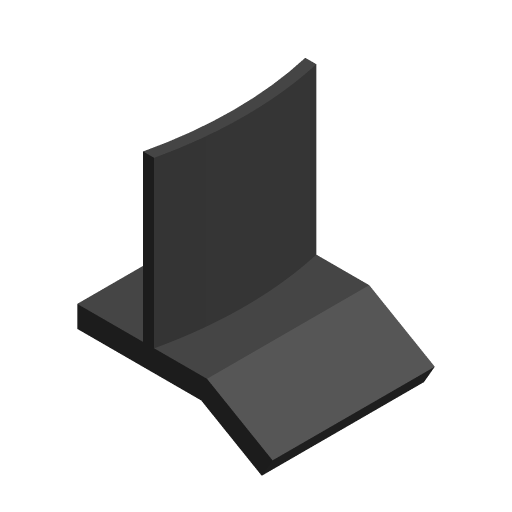
# Autodesk Inventor part: Camera retention
Saved by Autodesk Inventor 2024 (Build 280153000, 153)
## iProperties
Part Number: Camera retention
Material: Generic
Document SubType Name: Modeling
Designer: Jamie
Appearance: Default
Author: Jamie
Autodesk Inventor part; units mm, degrees
ref_plane "YZ Plane" through (0, 0, 0) normal (1, 0, 0) x (0, 1, 0)
ref_plane "XZ Plane" through (0, 0, 0) normal (0, 1, 0) x (-1, 0, 0)
ref_plane "XY Plane" through (0, 0, 0) normal (0, 0, 1) x (1, 0, 0)
sketch "Sketch3" plane through (0, 0, 0) normal (0, 1, 0) x (-1, 0, 0)
  circle A0 centre (0, 0) radius 33
  circle A1 centre (0, 0) radius 34
  line L0 (-30.4296, 7.5) -> (-38.9548, 7.5)
  line L1 (-38.9548, 7.5) -> (-38.9548, -7.5)
  line L2 (-38.9548, -7.5) -> (-30.4296, -7.5)
  line L3 (-30.4296, -7.5) -> (-30.4296, 7.5)
  point P0 (-33.1625, -7.5)
  point P1 (-32.1364, -7.5)
  point P2 (-32.1364, 7.5)
  point P3 (-33.1625, 7.5)
  dimension "d9" = 66
  dimension "d10" = 68
  dimension "d11" = 7.5
  dimension "d12" = 7.5
  constraints: 8 end point, 2 centre point, 2 coincident, 2 parallel, 1 horizontal, 1 perpendicular
  measures "d9" diameter of A0
  measures "d10" diameter of A1
  measures "d11" distance from line of point (0, 0) L0
  measures "d12" distance from line of point (0, 0) L2
extrude "Extrusion2" add sketch "Sketch3" along normal blind 15.25 contours A0 L2 A1 L0 picked at (-32.7342, -5.8399)
sketch "Sketch4" plane through (0, 0, 0) normal (0, -1, 0) x (1, 0, 0)
  line L0 (26.0495, 7.5) -> (38.0495, 7.5)
  line L1 (38.0495, 7.5) -> (38.0495, -7.5)
  line L2 (38.0495, -7.5) -> (26.0495, -7.5)
  line L3 (26.0495, -7.5) -> (26.0495, 7.5)
  line L4 (33.1625, -7.5) -> (32.1364, -7.5) projected
  line L5 (32.1364, 7.5) -> (33.1625, 7.5) projected
  point P0 (0, 0)
  point P1 (32.6495, -7.5)
  point P2 (32.6495, -7.5)
  dimension "d15" = 6.6
  dimension "d16" = 5.4
  dimension "d17" = 0
  dimension "d18" = 0
  constraints: 8 end point, 2 midpoint, 2 parallel, 1 horizontal, 1 perpendicular
  measures "d15" distance from line of L3 point (32.649, -7.5)
  measures "d16" distance from line of point (32.649, -7.5) L1
  measures "d17" distance between parallel lines of L4 L2
  measures "d18" distance between parallel lines of L5 L0
extrude "Extrusion3" add sketch "Sketch4" along normal blind 2
sketch "Sketch5" plane through (0, -2, 0) normal (0, -1, 0) x (1, 0, 0)
  circle A0 centre (29.0005, 0) radius 2
  line L0 (38.0495, 7.5) -> (26.0495, 7.5) projected
  line L1 (32.1364, 7.5) -> (33.1625, 7.5) projected
  point P0 (0, 0)
  point P1 (32.6495, 7.5)
  dimension "d21" = 4
  dimension "d22" = 7.5
  dimension "d23" = 3.649
  constraints: 1 centre point, 1 midpoint
  measures "d21" diameter of A0
  measures "d22" distance from line of L0 A0.centre
  measures "d23" horizontal distance of point (32.649, 7.5) A0.centre
extrude "Extrusion4" cut sketch "Sketch5" against normal blind 2
ref_plane "Work Plane1" through (38.0495, 0, -7.5) normal (0.5, 0.8660254, 0) x (0, 0, 1)
sketch "Sketch6" plane through (38.0495, 0, -7.5) normal (0.5, 0.8660254, 0) x (0, 0, 1)
  line L0 (15, 0) -> (0, 0)
  line L1 (0, 0) -> (0, 7)
  line L2 (0, 7) -> (15, 7)
  line L3 (15, 7) -> (15, 0)
  line L4 (0, 0) -> (15, 0) projected
  line L5 (15, 0) -> (15, -4.2322) projected
  line L6 (0, -4.2322) -> (0, 0) projected
  point P0 (7.5, -32.9518)
  point P1 (15, 3.5)
  dimension "d27" = 0
  dimension "d28" = 0
  dimension "d29" = 0
  dimension "d30" = 7
  constraints: 8 end point, 2 parallel, 1 horizontal, 1 midpoint, 1 perpendicular
  measures "d27" distance between parallel lines of L4 L0
  measures "d28" distance from line of L5 point (15, 3.5)
  measures "d29" distance between parallel lines of L6 L1
  measures "d30" distance of L0.end L1.end
extrude "Extrusion5" add sketch "Sketch6" against normal blind 2
sketch "Sketch7" plane through (37.0495, -1.7321, -7.5) normal (-0.5, -0.8660254, 0) x (0.8660254, -0.5, 0)
  circle A0 centre (5.0359, 4.5) radius 1
  circle A1 centre (5.0359, 10.5) radius 1
  ellipse E0 centre (-7.8367, 7.5) end of major axis (-7.8367, 9.5) minor radius 1.7321 projected
  line L0 (0.5359, 0) -> (0.5359, 15) projected
  point P0 (-32.9518, 7.5)
  dimension "d33" = 2
  dimension "d34" = 2
  dimension "d35" = 3
  dimension "d36" = 3
  dimension "d37" = 4.5
  dimension "d38" = 4.5
  constraints: 2 centre point
  measures "d33" diameter of A0
  measures "d34" diameter of A1
  measures "d35" vertical distance of E0.centre A0.centre
  measures "d36" vertical distance of A1.centre E0.centre
  measures "d37" distance from line of L0 A1.centre
  measures "d38" distance from line of L0 A0.centre
extrude "Extrusion6" add sketch "Sketch7" along normal blind 1.5 contours A0 | A1
body "Solid2"
